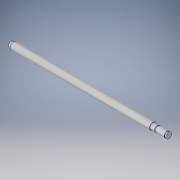
# Autodesk Inventor part: Saftey Axle
Saved by Autodesk Inventor 2019.4 (Build 234330000, 330)
## iProperties
Created: 2020-01-29
Part Number: Saftey Axle
Material: Aluminum 6061
Document SubType Name: Modeling
Designer: admin
Density: 2.7 g/cm^3
Appearance: Aluminum - Flat
Author: admin
Autodesk Inventor part; units mm, degrees
ref_plane "YZ Plane" through (0, 0, 0) normal (1, 0, 0) x (0, 1, 0)
ref_plane "XZ Plane" through (0, 0, 0) normal (0, 1, 0) x (-1, 0, 0)
ref_plane "XY Plane" through (0, 0, 0) normal (0, 0, 1) x (1, 0, 0)
sketch "Sketch1" plane through (0, 0, 0) normal (0, 0, 1) x (1, 0, 0)
  line L0 (0, 0) -> (0, 5)
  line L1 (0, 5) -> (4, 5)
  line L2 (4, 5) -> (4, 6)
  line L3 (4, 6) -> (250.6, 6)
  line L4 (250.6, 6) -> (250.6, 5)
  line L5 (250.6, 5) -> (258.6, 5)
  line L6 (258.6, 5) -> (258.6, 4.75)
  line L7 (258.6, 4.75) -> (259.7, 4.75)
  line L8 (259.7, 4.75) -> (259.7, 5)
  line L9 (259.7, 5) -> (275.7, 5)
  line L10 (275.7, 5) -> (275.7, 4.75)
  line L11 (275.7, 4.75) -> (276.8, 4.75)
  line L12 (276.8, 4.75) -> (276.8, 5)
  line L13 (276.8, 5) -> (278.8, 5)
  line L14 (278.8, 5) -> (278.8, 0)
  line L15 (278.8, 0) -> (0, 0)
  dimension "d0" = 4
  dimension "d1" = 5
  dimension "d2" = 6
  dimension "d3" = 1.1
  dimension "d4" = 1.1
  dimension "d5" = 0.25
  dimension "d6" = 2
  dimension "d7" = 16
  dimension "d8" = 246.6
  dimension "d9" = 8
  constraints: 32 end point, 11 perpendicular, 8 point on line, 1 vertical
  measures "d0" distance of L0.end L1.end
  measures "d1" distance between parallel lines of L15 L1
  measures "d2" distance between parallel lines of L15 L3
  measures "d3" distance of L6.end L7.end
  measures "d4" distance of L10.end L11.end
  measures "d5" distance of L5.end L6.end
  measures "d6" distance of L12.end L13.end
  measures "d7" distance of L8.end L9.end
  measures "d8" distance of L2.end L3.end
  measures "d9" distance of L4.end L5.end
revolve "Revolution1" add sketch "Sketch1" angle 360 about axis through (278.8, 0, 0) along (-1, 0, 0)
body "Solid1"
